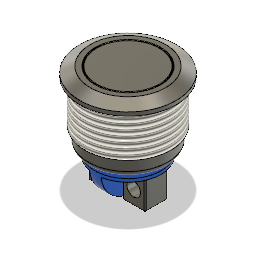
button (Autodesk Fusion 360 design; units mm, degrees)
Autodesk Fusion 360 part; units mm, degrees
note: some values were not read from the file. Chosen so that the rebuilt part matches the saved one: how an offset face is resized.
sketch "Sketch1" plane through (0, 0, 0) normal (0, 1, 0) x (1, 0, 0) in component "MetalBody"
  circle A0 centre (0, 0) radius 8.915
  dimension "d1" = 17.83
  measures "d1" diameter of A0
extrude "Extrude1" add sketch "Sketch1" along normal blind 0.7 makes body 1 in component "MetalBody"
extrude "Extrude2" add 1 faces at (-0.2221, 0.7, -2.5691) along direction (0, 1, 0) blind 1 on bodies 1 bodies 1 in component "MetalBody"
chamfer "Chamfer1" distance 2 distance2 1 1 edges at (-8.3117, 1.7, 3.2238) measured on face at (-0.2221, 1.7, -2.5691) on bodies 1 in component "MetalBody"
sketch "Sketch2" plane through (0, 1.7, 0) normal (0, 1, 0) x (-1, 0, 0) in component "MetalBody"
  circle A0 centre (0, 0) radius 6.915
  circle A1 centre (0, 0) radius 5.9
  dimension "d8" = 11.8
  measures "d8" diameter of A1
extrude "Extrude3" cut sketch "Sketch2" against normal through all contours A1 bodies 1 in component "MetalBody"
sketch "Sketch3" plane through (0, 0, 0) normal (0, 1, 0) x (1, 0, 0) in component "MetalBody"
  circle A0 centre (0, 0) radius 5.85
  dimension "d10" = 11.7
  measures "d10" diameter of A0
extrude "Extrude4" add sketch "Sketch3" along normal up to surface (1.7 mm away) separate body makes body 2 in component "MetalBody"
fillet "Fillet1" radius 0.1 2 edges at (5.5007, 1.7, 2.1335) (-5.4541, 1.7, -2.1155) on bodies 1 2 in component "MetalBody"
sketch "Sketch4" plane through (0, 0, 0) normal (0, -1, 0) x (1, 0, 0) in component "MetalBody"
  circle A0 centre (0, 0) radius 5.85
  circle A1 centre (0, 0) radius 7.9
  dimension "d14" = 15.8
  measures "d14" diameter of A1
extrude "Extrude5" add sketch "Sketch4" along normal blind 7.7 contours A0 | A1 bodies 1 2 in component "MetalBody"
sketch "Sketch5" plane through (0, -7.7, 0) normal (0, -1, 0) x (1, 0, 0) in component "MetalBody"
  circle A0 centre (0, 0) radius 7.9
  circle A1 centre (0, 0) radius 7.35
  dimension "d17" = 14.7
  measures "d17" diameter of A1
extrude "Extrude6" add sketch "Sketch5" along normal blind 3.22 contours A1 bodies 1 in component "MetalBody"
sketch "Sketch1 (2)" plane through (0, -10.92, 0) normal (0, -1, 0) x (1, 0, 0) in component "Plastic"
  circle A0 centre (0, 0) radius 7.35
  circle A1 centre (0, 0) radius 6.11
  dimension "d20" = 12.22
  measures "d20" diameter of A1
extrude "Extrude1'" add sketch "Sketch1 (2)" along normal blind 7 separate body contours A1 makes body 3 in component "Plastic"
fillet "Fillet1'" radius 6 1 edges at (-5.6965, -17.92, -2.2095) on bodies 3 in component "Plastic"
sketch "Sketch2 (2)" plane through (0, -17.92, 0) normal (0, -1, 0) x (1, 0, 0) in component "Plastic"
  circle A0 centre (0, 0) radius 0.11
  line L0 (1.05, 0) -> (-1.05, 0) construction
  line L1 (-1.05, -6.3688) -> (-6.6673, -6.3688)
  line L2 (-6.6673, -6.3688) -> (-6.6673, 6.5561)
  line L3 (-6.6673, 6.5561) -> (-1.05, 6.5561)
  line L4 (-1.05, 6.5561) -> (-1.05, -6.3688)
  line L5 (1.05, -6.3688) -> (7.2558, -6.3688)
  line L6 (7.2558, -6.3688) -> (7.2558, 6.5561)
  line L7 (7.2558, 6.5561) -> (1.05, 6.5561)
  line L8 (1.05, 6.5561) -> (1.05, -6.3688)
  dimension "d24" = 2.1
extrude "Extrude2'" cut sketch "Sketch2 (2)" against normal blind 5.4 contours L1 L2 L3 L4 | L5 L6 L7 L8 bodies 3 in component "Plastic"
sketch "Sketch6" plane through (0, -12.52, 0) normal (0, -1, 0) x (1, 0, 0) in component "MetalBody"
  arc A0 (-1.05, 5.9886) -> (-1.05, -5.9886) centre (0, 0) ccw
  line L0 (-1.05, -5.9886) -> (-1.05, 5.9886)
  line L1 (-5.25, 2.1) -> (-1.05, 2.1)
  line L2 (-1.05, 2.1) -> (-1.05, -2.1)
  line L3 (-1.05, -2.1) -> (-5.25, -2.1)
  line L4 (-5.25, -2.1) -> (-5.25, 2.1)
  line L5 (0, 0) -> (-1.05, 0) construction
  dimension "d27" = 4.2
  dimension "d28" = 4.2
extrude "Extrude7" add sketch "Sketch6" along normal blind 5.5 separate body contours L0 L1 L2 L3 L4 makes body 4 in component "MetalBody"
sketch "Sketch7" plane through (0, 0, -2.1) normal (0, 0, -1) x (-1, 0, 0) in component "MetalBody"
  line L0 (5.25, -12.52) -> (1.05, -12.52)
  line L1 (1.05, -12.52) -> (1.05, -18.02)
  line L2 (1.05, -18.02) -> (5.25, -18.02)
  line L3 (5.25, -18.02) -> (5.25, -12.52)
  line L4 (3.15, -12.52) -> (3.15, -18.02) construction
  circle A0 centre (3.15, -15.27) radius 1.25
  dimension "d31" = 2.5
  measures "d31" diameter of A0
extrude "Extrude8" cut sketch "Sketch7" against normal through all contours A0 bodies 4 in component "MetalBody"
chamfer "Chamfer2" distance 0.2 angle 45 8 edges at (-5.25, -15.27, 2.1) (-3.15, -18.02, 2.1) (-5.25, -18.02, 0) (-5.25, -15.27, -2.1) (-3.15, -18.02, -2.1) (-1.05, -15.27, -2.1) (-1.05, -18.02, 0) (-1.05, -15.27, 2.1) on bodies 4 in component "MetalBody"
mirror "Mirror1" about plane through (0, 0, 0) normal (1, 0, 0) of bodies 4 makes body 5 in component "MetalBody"
fillet "Fillet2" radius 1 1 edges at (-6.8526, -10.92, -2.6579) on bodies 1 in component "MetalBody"
thread "Thread1" "ISO Metric profile 16.0 M16x1 6g" major diameter 15.884 minor diameter 14.741 pitch 1 angle 60 resizes the face on face at (7.8902, -5.1333, -0.3938) on bodies 1 in component "MetalBody"
component "Button" placed x (1, 0, 0) y (0, 1, 0) z (0, 0, 1) at (0, 0, 0)
component "MetalBody" placed x (1, 0, 0) y (0, 1, 0) z (0, 0, 1) at (0, 0, 0) in component "Button"
component "Plastic" placed x (1, 0, 0) y (0, 1, 0) z (0, 0, 1) at (0, 0, 0) in component "Button"
equation "d15 = 9.4 mm - 1.7 mm"
